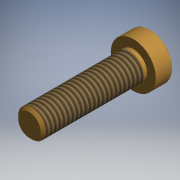
# Autodesk Inventor part: Zyl.Schr-M8x30_Stahl_X094960
Saved by Autodesk Inventor 2017.3 (Build 213256000, 256)
## iProperties
Part Number: Zyl.Schr-M8x30_Stahl_X094960
Material: Generic
Catalog Web Link: www.cadenas.de
Description: ZylSchraube DIN EN ISO 7984-Normalien
Vendor: ROSEKRIEGER
Document SubType Name: Modeling
Designer: partserver
Manufacturer: ROSEKRIEGER
Mass: 2.0543 g
Surface Area: 12.8932 cm^2
Volume: 2.0543 cm^3
Density: 1 g/cm^3
Appearance: PSOLRGB-203-152-72
Category: PARTsolutions
Company: ROSEKRIEGER
Title: Zyl.Schr-M8x30_Stahl_X094960
Author: Cadenas PARTsolutions
Comments: Normalien
PSOL_IDENT_0: {$CADENAS_DATA\23d-libs\rose_krieger\pool_normalien\schrauben_scheiben_muttern\zyl_isk_din7984.prj},
PSOL_IDENT_1: 219 {VTYP=3D},{NB=Zyl.Schr-M8x30_Stahl_X094960},{LINA=Zyl.Schr-M8x30_Stahl_X094960},{NN=ZylSchraube
PSOL_IDENT_2: DIN EN ISO 7984},{DATE=25.02.2021 18:00:30},{GEOMDATE=11.12.2020 13:50:00},{VERSION=},{LINEID=1110},
PSOL_IDENT_3: {WBVAR=},{WBNUMERIC=}  {NB=Zyl.Schr-M8x30_Stahl_X094960},{LINA=Zyl.Schr-M8x30_Stahl_X094960},{KT=DUM
PSOL_IDENT_4: MY},{IDNR=},{ARTIKEL=Zylinderschraube},{TYPE=M8},{FNENN=8.000},{L=30.000},{NORM=DIN7984},{NORMALT=DI
PSOL_IDENT_5: N7984},{BEST=X094960},{RKMATNR=X094960},{WERKSTOFFBEZ=Stahl},{WERKSTOFF=0},{OBERFLAECHE=1},{FKKL=8.8
PSOL_IDENT_6: },{KHOE=5.000},{KD=13.000},{B=29.000},{SW=5.000},{R=0.500},{TSS=5.000},{WARENNUMMER=73181569}
NB: Zyl.Schr-M8x30_Stahl_X094960
NN: ZylSchraube DIN EN ISO 7984
NT: Normalien
NBSYN: Zyl.Schr-$TYPE.x$L._$WERKSTOFFBEZ._$RKMATNR.
LINA: Zyl.Schr-M8x30_Stahl_X094960
CATALOG: RK Rose+Krieger
ARTIKEL: Zylinderschraube
TYPE: M8
FNENN: 8
L: 30
NORM: DIN7984
NORMALT: DIN7984
BEST: X094960
RKMATNR: X094960
WERKSTOFFBEZ: Stahl
WERKSTOFF: 0
OBERFLAECHE: 1
FKKL: 8.8
KHOE: 5
KD: 13
B: 29
SW: 5
R: 0.5
TSS: 5
WARENNUMMER: 73181569
SUPPLIER: ROSEKRIEGER
ARTICLENO: Zyl.Schr-M8x30_Stahl_X094960
BOMINFO: Zyl.Schr-M8x30_Stahl_X094960
CREATOR: CADENAS GmbH
Autodesk Inventor part; units mm, degrees
ref_plane "YZ Plane" through (0, 0, 0) normal (1, 0, 0) x (0, 1, 0)
ref_plane "XZ Plane" through (0, 0, 0) normal (0, 1, 0) x (-1, 0, 0)
ref_plane "XY Plane" through (0, 0, 0) normal (0, 0, 1) x (1, 0, 0)
sketch "Skizze_1" plane through (0, 0, 0) normal (0, 0, 1) x (1, 0, 0)
  line L0 (0, -30) -> (0, 0)
  line L1 (0, 0) -> (4, 0)
  line L2 (4, 0) -> (4, -29.233)
  line L3 (4, -29.233) -> (3.233, -30)
  line L4 (3.233, -30) -> (0, -30)
  line L5 (0, -30) -> (0, 0)
  constraints: 12 end point
revolve "Revolution1" add sketch "Skizze_1" angle 360 about axis through (0, -30, 0) along (0, -1, 0)
thread "Thread1" size "M8x1.25" class "6g" standard "ISO Metric profile" length 29 offset 1
sketch "Skizze_2" plane through (0, 0, 0) normal (0, 0, 1) x (1, 0, 0)
  line L0 (0, 0) -> (0, 5)
  line L1 (0, 5) -> (6, 5)
  arc A0 (6.5, 4.5) -> (6, 5) centre (6, 4.5) ccw
  line L2 (6.5, 4.5) -> (6.5, 0)
  line L3 (6.5, 0) -> (0, 0)
  line L4 (0, 0) -> (0, 5)
  constraints: 10 end point, 2 point on circle, 1 centre point
revolve "Revolution2" add sketch "Skizze_2" angle 360 about axis through (0, 0, 0) along (0, -1, 0)
sketch "Skizze_3" plane through (0, 5, 0) normal (0, 1, 0) x (1, 0, 0)
  line L0 (-2.5, -1.4434) -> (0, -2.8868)
  line L1 (0, -2.8868) -> (2.5, -1.4434)
  line L2 (2.5, -1.4434) -> (2.5, 1.4434)
  line L3 (2.5, 1.4434) -> (0, 2.8868)
  line L4 (0, 2.8868) -> (-2.5, 1.4434)
  line L5 (-2.5, 1.4434) -> (-2.5, -1.4434)
  constraints: 12 end point
extrude "Extrusion1" cut sketch "Skizze_3" against normal blind 5
ref_plane "EP_XY" through (0, 0, 0) normal (0, 1, 0) x (1, 0, 0)
ref_plane "EP_YZ" through (0, 0, 0) normal (1, 0, 0) x (0, 0, -1)
ref_plane "EP_ZX" through (0, 0, 0) normal (0, 0, -1) x (0, 1, 0)
ref_plane "EP_Schraube_XY" through (0, 0, 0) normal (0, 1, 0) x (1, 0, 0)
ref_plane "EP_Schraube_YZ" through (0, 0, 0) normal (1, 0, 0) x (0, 0, -1)
ref_plane "EP_Schraube_ZX" through (0, 0, 0) normal (0, 0, -1) x (0, 1, 0)
body "Solid1"
